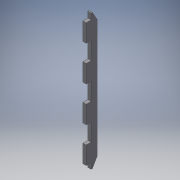
# Autodesk Inventor part: TrayPanelH
Saved by Autodesk Inventor 2017 (Build 210142000, 142)
## iProperties
Created: 2019-06-23
Part Number: TrayPanelH
Material: Generic
Document SubType Name: Modeling
Designer: DDeGo
Density: 1 g/cm^3
Appearance: Default
Author: DDeGo
Autodesk Inventor part; units mm, degrees
ref_plane "YZ Plane" through (0, 0, 0) normal (1, 0, 0) x (0, 1, 0)
ref_plane "XZ Plane" through (0, 0, 0) normal (0, 1, 0) x (-1, 0, 0)
ref_plane "XY Plane" through (0, 0, 0) normal (0, 0, 1) x (1, 0, 0)
sketch "Sketch1" plane through (0, 0, 0) normal (1, 0, 0) x (0, 1, 0)
  line L0 (0, 0) -> (0, 115)
  line L1 (0, 115) -> (1, 115)
  line L2 (1, 115) -> (5, 108.0718)
  line L3 (5, 108.0718) -> (5, 6.9282)
  line L4 (5, 6.9282) -> (1, 0)
  line L5 (1, 0) -> (0, 0)
  line L6 (1, 115) -> (1, 0) construction
  dimension "d0" = 1
  dimension "d1" = 4
  dimension "d2" = 30
  dimension "d3" = 115
  constraints: 14 end point, 2 parallel, 2 vertical, 1 equal length, 1 perpendicular
  measures "d0" distance between parallel lines of L0 L6
  measures "d1" distance between parallel lines of L3 L6
  measures "d2" angle of L6 L4
  measures "d3" distance between parallel lines of L1 L5
extrude "Extrusion1" add sketch "Sketch1" along normal blind 2.75
sketch "Sketch2" plane through (2.75, 0, 0) normal (1, 0, 0) x (0, 0, -1)
  line L0 (-115, 0) -> (0, 0) projected
  line L1 (-110, 0) -> (-94.85, 0)
  line L2 (-94.85, 0) -> (-94.85, -4.2)
  line L3 (-94.85, -4.2) -> (-110, -4.2)
  line L4 (-110, -4.2) -> (-110, 0)
  line L5 (-80, 0) -> (-64.85, 0)
  line L6 (-64.85, 0) -> (-64.85, -4.2)
  line L7 (-64.85, -4.2) -> (-80, -4.2)
  line L8 (-80, -4.2) -> (-80, 0)
  line L9 (-50, 0) -> (-34.85, 0)
  line L10 (-34.85, 0) -> (-34.85, -4.2)
  line L11 (-34.85, -4.2) -> (-50, -4.2)
  line L12 (-50, -4.2) -> (-50, 0)
  line L13 (-20, 0) -> (-4.85, 0)
  line L14 (-4.85, 0) -> (-4.85, -4.2)
  line L15 (-4.85, -4.2) -> (-20, -4.2)
  line L16 (-20, -4.2) -> (-20, 0)
  dimension "d6" = 15.15
  dimension "d7" = 15.15
  dimension "d8" = 15.15
  dimension "d9" = 15.15
  dimension "d10" = 4.2
  dimension "d11" = 5
  dimension "d12" = 30
  dimension "d13" = 30
  dimension "d14" = 30
  constraints: 32 end point, 8 parallel, 7 point on line, 4 horizontal, 4 perpendicular
  measures "d6" distance of L2.end L3.end
  measures "d7" distance of L6.end L7.end
  measures "d8" distance of L10.end L11.end
  measures "d9" distance of L14.end L15.end
  measures "d10" distance of L3.end L1.start
  measures "d11" horizontal distance of L0.start L3.end
  measures "d12" distance of L7.end L3.end
  measures "d13" distance of L11.end L7.end
  measures "d14" distance of L11.end L15.end
extrude "Extrusion2" add sketch "Sketch2" against normal up to surface (2.75 mm away)
equation "\"d7\" = d6"
equation "\"d8\" = d6"
equation "\"d9\" = d6"
equation "\"d13\" = d12"
equation "\"d14\" = d12"
body "Solid1"
